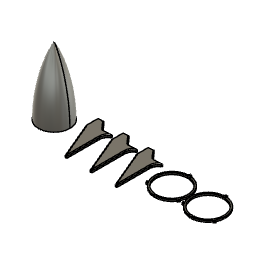
Water Rocket Comps v1 v2 (Autodesk Fusion 360 design; units mm, degrees)
Autodesk Fusion 360 part; units mm, degrees
sketch "Sketch1" plane through (0, 0, 0) normal (0, 0, 1) x (1, 0, 0)
  line L0 (0, 0) -> (0, 107.95)
  line L1 (0, 0) -> (25.4, 0)
  line L2 (0, 107.95) -> (0.635, 107.95)
  line L3 (0.635, 107.95) -> (3.81, 104.14)
  line L4 (3.81, 104.14) -> (17.78, 76.2)
  line L5 (17.78, 76.2) -> (25.4, 38.1)
  line L6 (25.4, 38.1) -> (25.4, 0)
  spline S0 degree 4 poles (0.635, 107.95) (3.81, 104.14) (17.78, 76.2) (25.4, 38.1) (25.4, 0) knots 0 0 0 0 0 1 1 1 1 1
  dimension "d1" = 107.95
  dimension "d2" = 25.4
  dimension "d3" = 0.635
  constraint coincident L0.start L1.start
  constraint vertical L0
  constraint perpendicular L0 L1
  constraint perpendicular L0 L2
  measures "d1" distance of L0.start L0.end
  measures "d2" distance of L0.start L1.end
  measures "d3" distance of L0.end L2.end
revolve "Revolve1" add sketch "Sketch1" angle 360 about axis through (0, 0, 0) along (0, 1, 0) contours L0 L1 L2 S0 makes body 1
hole "Hole1" at (0, 0, 0) direction (0, 1, 0) diameter 22.86 depth 50.8 tip angle 118 bodies 1
sketch "Sketch2" plane through (0, 0, 0) normal (0, 1, 0) x (1, 0, 0)
  line L0 (104.14, -45.72) -> (104.14, 7.62)
  line L1 (104.14, -45.72) -> (101.6, -45.72)
  line L2 (101.6, -45.72) -> (76.2, 14.3164)
  line L3 (76.2, 14.3164) -> (76.2, 33.02)
  line L4 (76.2, 33.02) -> (85.5133, 33.02)
  line L5 (85.5133, 33.02) -> (96.52, 20.32)
  line L6 (96.52, 20.32) -> (111.76, 20.32)
  arc A0 (111.76, 20.32) -> (104.14, 7.62) centre (118.5333, 7.62) ccw
  constraint vertical L0
  constraint perpendicular L0 L1
  constraint parallel L0 L3
  constraint perpendicular L3 L4
  constraint perpendicular L3 L6
  constraint tangent L0 A0
extrude "Extrude1" add sketch "Sketch2" along normal blind 5.08 separate body makes body 2
fillet "Fillet1" radius 1.27 15 edges at (104.14, 5.08, 19.05) (106.1912, 5.08, -15.0253) (104.14, 5.08, -20.32) (91.0167, 5.08, -26.67) (80.8567, 5.08, -33.02) (76.2, 5.08, -23.6682) (88.9, 5.08, 15.7018) (104.14, 0, 19.05) (106.1912, 0, -15.0253) (88.9, 0, 15.7018) (102.87, 0, 45.72) (76.2, 0, -23.6682) (80.8567, 0, -33.02) (91.0167, 0, -26.67) (104.14, 0, -20.32) on bodies 2
copy_body "CopyPasteBodies1" bodies 2 makes body 3
move_body "Move1" bodies 3 to x (1, 0, 0) y (0, 1, 0) z (0, 0, 1) at (40.64, 0, 0)
copy_body "CopyPasteBodies2" bodies 3 makes body 4
move_body "Move2" bodies 4 to x (1, 0, 0) y (0, 1, 0) z (0, 0, 1) at (40.64, 0, 0)
sketch "Sketch3" plane through (0, 0, 0) normal (0, 1, 0) x (1, 0, 0)
  circle A0 centre (228.6, 0) radius 25.4
  line L0 (226.9228, 30.4161) -> (228.1928, 30.4161)
  line L1 (228.1928, 30.4161) -> (228.1928, 27.937)
  line L2 (226.9228, 27.8876) -> (226.9228, 30.4161)
  line L3 (228.9848, 30.4161) -> (230.2295, 30.4161)
  line L4 (230.2295, 30.4161) -> (230.2295, 27.8924)
  line L5 (228.9848, 27.9374) -> (228.9848, 30.4161)
  arc A1 (228.9848, 27.9374) -> (228.1928, 27.937) centre (228.6, 0) ccw
  line L6 (202.4625, -15.5607) -> (204.6094, -14.3211)
  line L7 (203.0975, -16.6605) -> (202.4625, -15.5607)
  line L8 (205.2872, -15.3963) -> (203.0975, -16.6605)
  line L9 (204.2132, -13.6354) -> (202.0665, -14.8748)
  line L10 (202.0665, -14.8748) -> (201.4442, -13.7969)
  line L11 (201.4442, -13.7969) -> (203.6297, -12.535)
  line L12 (255.1447, -14.8554) -> (252.9978, -13.6159)
  line L13 (255.7797, -13.7556) -> (255.1447, -14.8554)
  line L14 (253.5899, -12.4913) -> (255.7797, -13.7556)
  line L15 (252.6021, -14.3019) -> (254.7487, -15.5413)
  line L16 (254.7487, -15.5413) -> (254.1264, -16.6192)
  line L17 (254.1264, -16.6192) -> (251.9408, -15.3574)
  arc A2 (226.9228, 27.8896) -> (203.6297, -12.535) centre (228.6, 0) ccw
  arc A3 (204.2132, -13.6354) -> (204.6094, -14.3211) centre (228.6, 0) ccw
  arc A4 (205.2855, -15.3973) -> (251.9408, -15.3574) centre (228.6, 0) ccw
  arc A5 (252.6021, -14.3019) -> (252.9978, -13.6159) centre (228.6, 0) ccw
  arc A6 (253.5917, -12.4923) -> (230.2295, 27.8924) centre (228.6, 0) ccw
  dimension "d12" = 50.8
  dimension "d14" = 1.27
  dimension "d16" = 360
  constraint horizontal L0
  constraint vertical L1
  constraint vertical L2
  constraint horizontal L3
  constraint vertical L4
  constraint vertical L5
  constraint concentric A0 A1
  constraint coincident L2 A2.start
  constraint concentric A1 A2
  constraint concentric A2 A3
  constraint coincident L8 A4.start
  constraint concentric A3 A4
  constraint concentric A4 A5
  constraint coincident L14 A6.start
  constraint concentric A5 A6
  measures "d12" diameter of A0
  measures "d14" distance of L0.start L0.end
extrude "Extrude2" add sketch "Sketch3" along normal blind 2.54 separate body makes body 5
copy_body "CopyPasteBodies3" bodies 5 makes body 6
move_body "Move3" bodies 6 to x (1, 0, 0) y (0, 1, 0) z (0, 0, 1) at (58.42, 0, 0)
move_body "Move4" bodies 1 to x (1, 0, 0) y (0, 1, 0) z (0, 0, 1) at (38.1, 0, 0)
sketch "Sketch4" plane through (0, 0, 0) normal (0, 1, 0) x (1, 0, 0)
